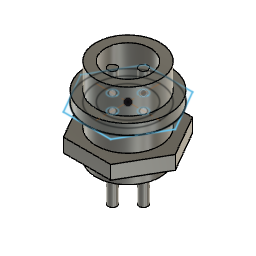
Device-TempHum-NodeController v13 (Autodesk Fusion 360 archive; units mm, degrees)
design "4pin round connector"
Autodesk Fusion 360 part; units mm, degrees
sketch "Sketch1" plane through (0, 0, 0) normal (0, 0, 1) x (1, 0, 0) in component "Socket"
  circle A0 centre (0, 0) radius 5.85
  line L0 (0, 5.85) -> (0, -5.85)
  line L1 (-5.85, 0) -> (5.85, 0)
  circle A1 centre (0, 2.85) radius 0.8
  circle A2 centre (0, -2.85) radius 0.8
  circle A3 centre (2.85, 0) radius 0.8
  circle A4 centre (-2.85, 0) radius 0.8
  circle A5 centre (0, 0) radius 7.5
  circle A6 centre (0, 0) radius 4.1
  line L2 (4.3301, -7.5) -> (8.6603, 0)
  line L3 (8.6603, 0) -> (4.3301, 7.5)
  line L4 (4.3301, 7.5) -> (-4.3301, 7.5)
  line L5 (-4.3301, 7.5) -> (-8.6603, 0)
  line L6 (-8.6603, 0) -> (-4.3301, -7.5)
  line L7 (-4.3301, -7.5) -> (4.3301, -7.5)
  dimension "d1" = 11.7
  dimension "d2" = 1.6
  dimension "d3" = 3
  dimension "d4" = 1.6
  dimension "d5" = 3
  dimension "d6" = 15
  dimension "d11" = -1.75
  dimension "d19" = 7.5
  constraint coincident A0.centre A5.centre
  constraint coincident A0 L0.start
  constraint coincident A0 L0.end
  constraint vertical L0
  constraint coincident A0 L1.start
  constraint coincident A0 L1.end
  constraint perpendicular L0 L1
  constraint coincident L0 A1.centre
  constraint symmetric L1 A1 A2
  constraint symmetric L0 A3 A4
  constraint concentric A0 A5
  measures "d1" diameter of A0
  measures "d2" diameter of A1
  measures "d3" distance of L0.start A1.centre
  measures "d4" diameter of A3
  measures "d5" distance of L1.end A3.centre
  measures "d6" diameter of A5
  measures "d19" distance of A0.centre L7
extrude "Extrude1" add sketch "Sketch1" along normal blind 1.9 contours A5 makes body 1 in component "Socket"
extrude "Extrude2" add sketch "Sketch1" along normal blind 6.5 contours A0 L0 L1 A6 | A0 L0 L1 A6 | A0 L0 L1 A6 | A0 L0 L1 A6 bodies 1 in component "Socket"
extrude "Extrude3" add sketch "Sketch1" along normal blind 4 separate body contours L1 A3 | L1 A3 | L0 A1 | L0 A1 | L0 A2 | L0 A2 | L1 A4 | L1 A4 makes body 2 at (3.649, -0.0399, 1.3333) makes body 3 at (-2.051, -0.0399, 1.3333) makes body 4 at (0.796, 2.9297, 2.6667) makes body 5 at (0.796, -2.7703, 2.6667) in component "Socket"
extrude "Extrude4" add sketch "Sketch1" against normal blind 9 contours A0 L0 L1 A6 | A0 L0 L1 A6 | A0 L0 L1 A6 | A0 L0 L1 A6 | L0 L1 A2 A3 A6 | L0 L1 A1 A3 A6 | L0 L1 A1 A4 A6 | L0 L1 A2 A4 A6 bodies 1 2 3 4 5 in component "Socket"
extrude "Extrude5" add sketch "Sketch1" against normal blind 14.75 separate body contours L1 A3 | L1 A3 | L0 A1 | L0 A1 | L0 A2 | L0 A2 | L1 A4 | L1 A4 makes body 6 at (3.649, -0.0399, -9.8333) makes body 7 at (-2.051, -0.0399, -9.8333) makes body 8 at (0.796, -2.7703, -4.9167) makes body 9 at (0.796, 2.9297, -4.9167) in component "Socket"
extrude "Extrude6" add sketch "Sketch1" 1 faces at (6.9221, -0.3726, 0) against normal blind 2.5 from surface at -4 separate body contours A5 L2 L3 | A5 L3 L4 | A5 L2 L7 | A5 L4 L5 | A5 L6 L7 | A5 L5 L6 on bodies 1 makes body 10 in component "Socket"
component "Socket" placed x (1, 0, 0) y (0, 1, 0) z (0, 0, 1) at (0, 0, 0)
equation "d17 = -9.00 mm + -5.75 mm"
